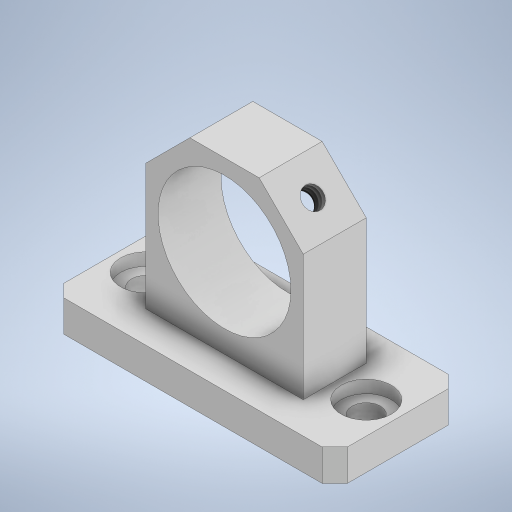
# Autodesk Inventor part: ADAPTER_I-355-03
Saved by Autodesk Inventor 2024.2 (Build 282272000, 272)
## iProperties
Created: 2024-01-09
Part Number: ADAPTER_I-355-03
Material: Generic
Document SubType Name: Modeling
Designer: fabig
Density: 1 g/cm^3
Appearance: Default
Author: fabig
Autodesk Inventor part; units mm, degrees
ref_plane "YZ Plane" through (0, 0, 0) normal (1, 0, 0) x (0, 1, 0)
ref_plane "XZ Plane" through (0, 0, 0) normal (0, 1, 0) x (-1, 0, 0)
ref_plane "XY Plane" through (0, 0, 0) normal (0, 0, 1) x (1, 0, 0)
sketch "Sketch2" plane through (0, 0, 0) normal (0, 1, 0) x (-1, 0, 0)
  line L0 (-22.5, 10) -> (22.5, 10)
  line L1 (22.5, 10) -> (22.5, -10)
  line L2 (22.5, -10) -> (-22.5, -10)
  line L3 (-22.5, -10) -> (-22.5, 10)
  line L4 (-22.5, 10) -> (22.5, -10) construction
  line L5 (22.5, 10) -> (-22.5, -10) construction
  point P0 (0, 0)
  dimension "d0" = 45
  dimension "d1" = 20
  constraints: 12 end point, 2 midpoint, 2 parallel, 1 horizontal, 1 perpendicular
  measures "d0" distance of L1.end L2.end
  measures "d1" distance of L0.end L1.end
extrude "Extrusion1" add sketch "Sketch2" along normal blind 5
sketch "Sketch3" plane through (0, 5, 0) normal (0, 1, 0) x (1, 0, 0)
  line L0 (12.5, -5) -> (-12.5, -5)
  line L1 (-12.5, -5) -> (-12.5, 5)
  line L2 (-12.5, 5) -> (12.5, 5)
  line L3 (12.5, 5) -> (12.5, -5)
  line L4 (12.5, -5) -> (-12.5, 5) construction
  line L5 (-12.5, -5) -> (12.5, 5) construction
  point P0 (0, 0)
  dimension "d4" = 25
  dimension "d5" = 10
  constraints: 12 end point, 2 midpoint, 2 parallel, 1 horizontal, 1 perpendicular
  measures "d4" distance of L1.end L2.end
  measures "d5" distance of L0.end L1.end
extrude "Extrusion2" add sketch "Sketch3" along normal blind 27
sketch "Sketch4" plane through (12.5, 5, -5) normal (0, 0, -1) x (-1, 0, 0)
  line L0 (35, 0) -> (-10, 0) construction
  line L1 (12.5, 0) -> (12.5, 14.05) construction
  circle A0 centre (12.5, 14.05) radius 10.55
  point P0 (12.5, -5)
  dimension "d8" = 14.05
  dimension "d9" = 21.1
  constraints: 2 end point, 1 centre point, 1 coincident, 1 midpoint, 1 vertical
  measures "d8" distance of L1.start L1.end
  measures "d9" diameter of A0
extrude "Extrusion3" cut sketch "Sketch4" against normal up to surface (10 mm away)
chamfer "Chamfer1" distance 7 angle 45 2 edges at (12.5, 32, 0) (-12.5, 32, 0)
sketch "Sketch6" plane through (5.5, 32, -5) normal (0.7071, 0.7071, 0) x (-0.7071, 0.7071, 0)
  line L0 (0, 0) -> (0, 10) construction
  line L1 (-9.8995, 10) -> (-9.8995, 0) construction
  line L2 (0, 10) -> (-9.8995, 0) construction
  line L3 (-9.8995, 0) -> (-9.8995, 10) construction
  line L4 (-9.8995, 10) -> (0, 0) construction
  line L5 (0, 0) -> (-4.9497, 5) construction
  point P0 (-18.7383, 5)
  constraints: 8 end point, 1 collinear, 1 midpoint
hole "Hole1" at (9, 28.5, 0) direction (-0.7071, -0.7071, 0) diameter 3.302 depth 12.3 thread size "8-32 UNC" class "2B" standard "ANSI Unified Screw Threads"
sketch "Sketch7" plane through (-5.5, 32, -5) normal (-0.7071, 0.7071, 0) x (-0.7071, -0.7071, 0)
  line L0 (0, 10) -> (0, 0) construction
  line L1 (24.0416, 0) -> (9.8995, 0) construction
  line L2 (0, 10) -> (9.8995, 0) construction
  line L3 (9.8995, 0) -> (4.9497, 5) construction
  point P0 (18.7383, 5)
  constraints: 4 end point, 1 midpoint
hole "Hole2" at (-9, 28.5, 0) direction (0.7071, -0.7071, 0) diameter 3.302 depth 12.3 thread size "8-32 UNC" class "2B" standard "ANSI Unified Screw Threads"
sketch "Sketch13" plane through (0, 5, 0) normal (0, 1, 0) x (1, 0, 0)
  line L0 (-22.5, 10) -> (-22.5, -10) construction
  line L1 (-22.5, 0) -> (-17.5, 0) construction
  line L2 (22.5, -10) -> (22.5, 10) construction
  line L3 (22.5, 0) -> (17.5, 0) construction
  circle A0 centre (17.5, 0) radius 4
  circle A1 centre (-17.5, 0) radius 4
  point P0 (0, 0)
  dimension "d69" = 5
  dimension "d70" = 5
  dimension "d71" = 8
  dimension "d72" = 8
  constraints: 4 end point, 2 centre point, 2 coincident, 2 horizontal, 2 midpoint
  measures "d69" distance of L1.start L1.end
  measures "d70" distance of L3.start L3.end
  measures "d71" diameter of A0
  measures "d72" diameter of A1
extrude "Extrusion8" cut sketch "Sketch13" against normal blind 2
sketch "Sketch14" plane through (0, 5, 0) normal (0, 1, 0) x (1, 0, 0)
  circle A0 centre (17.5, 0) radius 4 projected
  circle A1 centre (17.5, 0) radius 2.25
  circle A2 centre (-17.5, 0) radius 4 projected
  circle A3 centre (-17.5, 0) radius 2.25
  point P0 (0, 0)
  dimension "d75" = 4.5
  constraints: 2 centre point, 2 coincident
  measures "d75" diameter of A1
extrude "Extrusion9" cut sketch "Sketch14" against normal through all contours A1 | A3
sketch "Sketch15" plane through (0, 0, 0) normal (0, -1, 0) x (1, 0, 0)
  circle A0 centre (-17.5, 0) radius 2.25 construction
  line L0 (-17.5, 0) -> (-12.5, 0) construction
  circle A1 centre (17.5, 0) radius 2.25 construction
  line L1 (17.5, 0) -> (13, 0) construction
  circle A2 centre (-12.5, 0) radius 1.005
  circle A3 centre (13, 0) radius 1.005
  line L2 (13, 0) -> (12, 0) construction
  circle A4 centre (12, 0) radius 1.005
  line L3 (12, 1.005) -> (13, 1.005)
  line L4 (13, -1.005) -> (12, -1.005)
  point P0 (0, 0)
  dimension "d78" = 5
  dimension "d79" = 4.5
  dimension "d80" = 2.01
  dimension "d81" = 2.01
  dimension "d82" = 1
  dimension "d83" = 2.01
  constraints: 10 end point, 4 point on circle, 4 tangent, 3 centre point, 3 coincident, 3 horizontal
  measures "d78" distance of L0.start L0.end
  measures "d79" distance of L1.start L1.end
  measures "d80" diameter of A2
  measures "d81" diameter of A3
  measures "d82" distance of L2.start L2.end
  measures "d83" diameter of A4
extrude "Extrusion10" cut sketch "Sketch15" against normal blind 2.1
chamfer "Chamfer3" distance 2 angle 45 4 edges at (-22.5, 2.5, 10) (22.5, 2.5, 10) (-22.5, 2.5, -10) (22.5, 2.5, -10)
body "Solid1"
